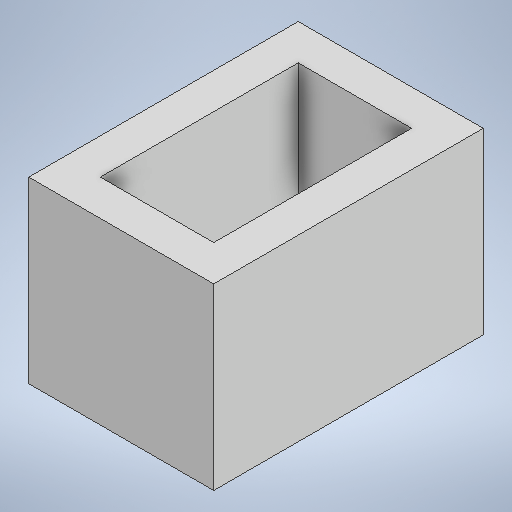
# Autodesk Inventor part: SwitchHolder
Saved by Autodesk Inventor 2027 (Build 310192060, 192F)
## iProperties
Created: 2026-07-14
Part Number: SwitchHolder
Material: Generic
Document SubType Name: Modeling
Designer: 13129
Density: 1 g/cm^3
Appearance: Default
Author: 13129
Autodesk Inventor part; units mm, degrees
ref_plane "YZ Plane" through (0, 0, 0) normal (1, 0, 0) x (0, 1, 0)
ref_plane "XZ Plane" through (0, 0, 0) normal (0, 1, 0) x (-1, 0, 0)
ref_plane "XY Plane" through (0, 0, 0) normal (0, 0, 1) x (1, 0, 0)
sketch "Sketch1" plane through (0, 0, 0) normal (0, 1, 0) x (-1, 0, 0)
  line L0 (8.05, -14.05) -> (-8.05, -14.05)
  line L1 (-8.05, -14.05) -> (-8.05, 14.05)
  line L2 (-8.05, 14.05) -> (8.05, 14.05)
  line L3 (8.05, 14.05) -> (8.05, -14.05)
  line L4 (13.13, -19.13) -> (-13.13, -19.13)
  line L5 (-13.13, -19.13) -> (-13.13, 19.13)
  line L6 (-13.13, 19.13) -> (13.13, 19.13)
  line L7 (13.13, 19.13) -> (13.13, -19.13)
  point P0 (0, 0)
  point P1 (8.05, 0)
  point P2 (0, -14.05)
  dimension "d0" = 16.1
  dimension "d1" = 28.1
  dimension "d2" = 5.08
  dimension "d3" = 5.08
  dimension "d4" = 5.08
  dimension "d5" = 5.08
  constraints: 16 end point, 4 parallel, 2 horizontal, 2 midpoint, 2 perpendicular, 1 horizontal alignment, 1 vertical alignment
  measures "d0" distance of L1.end L2.end
  measures "d1" distance of L0.end L1.end
  measures "d2" distance between parallel lines of L4 L0
  measures "d3" distance between parallel lines of L5 L1
  measures "d4" distance between parallel lines of L2 L6
  measures "d5" distance between parallel lines of L7 L3
extrude "Extrusion1" add sketch "Sketch1" along normal blind 25.4
body "Solid1"
